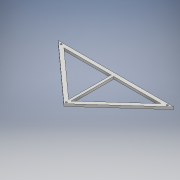
# Autodesk Inventor part: Down base
Saved by Autodesk Inventor 2018 (Build 220112000, 112)
## iProperties
Created: 2019-11-10
Part Number: Down base
Material: Типовые
Document SubType Name: Modeling
Designer: cosko
Density: 1 g/cm^3
Appearance: По умолчанию
Author: cosko
Autodesk Inventor part; units mm, degrees
ref_plane "YZ Plane" through (0, 0, 0) normal (1, 0, 0) x (0, 1, 0)
ref_plane "XZ Plane" through (0, 0, 0) normal (0, 1, 0) x (-1, 0, 0)
ref_plane "XY Plane" through (0, 0, 0) normal (0, 0, 1) x (1, 0, 0)
sketch "Эскиз1" plane through (0, 0, 0) normal (0, 0, 1) x (1, 0, 0)
  line L0 (-100, -100) -> (100, -100)
  line L1 (100, -100) -> (100, 100)
  line L2 (100, 100) -> (-100, 100)
  line L3 (-100, 100) -> (-100, -100)
  line L4 (-100, -100) -> (100, 100) construction
  line L5 (100, -100) -> (-100, 100) construction
  point P0 (0, 0)
  dimension "d0" = 200
  dimension "d1" = 200
  constraints: 12 end point, 2 midpoint, 2 parallel, 1 horizontal, 1 perpendicular
  measures "d0" distance of L2.end L1.end
  measures "d1" distance of L1.end L0.end
extrude "Выдавливание1" add sketch "Эскиз1" along normal blind 3
sketch "Эскиз2" plane through (0, 0, 3) normal (0, 0, 1) x (1, 0, 0)
  line L0 (-100, -100) -> (100, -100) projected
  line L1 (100, -100) -> (100, 100) projected
  line L2 (100, 100) -> (-100, 100) projected
  line L3 (-100, 100) -> (-100, -100) projected
  line L4 (-100, 100) -> (-90, 100) construction
  line L5 (-100, -100) -> (100, -100) construction
  line L6 (100, -100) -> (90, -100) construction
  line L7 (-90, 100) -> (-90, 90) construction
  line L8 (100, 100) -> (-100, 100) construction
  line L9 (-90, 100) -> (-80, 100) construction
  line L10 (90, -100) -> (90, -90) construction
  line L11 (-90, 90) -> (90, 90) construction
  line L12 (90, 90) -> (90, -90) construction
  line L13 (90, -90) -> (-90, -90) construction
  line L14 (-90, -90) -> (-90, 90) construction
  point P0 (0, 0)
  dimension "d4" = 10
  dimension "d5" = 10
  dimension "d6" = 10
  dimension "d7" = 270
  dimension "d8" = 10
  constraints: 18 end point, 3 perpendicular, 2 horizontal, 2 parallel, 2 point on line, 1 vertical
  measures "d4" distance of L2.end L4.end
  measures "d5" distance of L0.end L6.end
  measures "d6" distance of L4.end L7.end
  measures "d8" distance of L6.end L10.end
sketch "Эскиз3" plane through (0, 0, 0) normal (0, 0, -1) x (-1, 0, 0)
  line L0 (-90, -90) -> (90, -90) construction
  line L1 (90, -90) -> (90, 90) construction
  line L2 (90, 90) -> (-90, 90) construction
  line L3 (100, -100) -> (-100, -100) projected
  line L4 (-100, -100) -> (-100, 100) projected
  line L5 (-100, 100) -> (100, 100) projected
  line L6 (100, 100) -> (100, -100) projected
  line L7 (-90, 90) -> (-90, -90) construction
  point P0 (0, 0)
sketch "Эскиз4" plane through (0, 0, 0) normal (0, 0, -1) x (-1, 0, 0)
  line L0 (90, -90) -> (90, 90) construction
  line L1 (-90, -90) -> (90, -90) construction
  line L2 (90, -90) -> (80, -90) construction
  line L3 (80, -90) -> (80, -57.8) construction
  line L4 (80, -57.8) -> (69, -57.8) construction
  line L5 (69, -57.8) -> (69, -90) construction
  line L6 (74.5, -90) -> (74.5, -58.2367) construction
  line L7 (80, -73.9) -> (69, -73.9) construction
  line L8 (74.5, -90) -> (74.5, -82.5) construction
  circle A0 centre (74.5, -82.5) radius 2
  line L9 (74.5, -82.5) -> (74.5, -75) construction
  line L10 (74.5, -75) -> (74.5, -67.5) construction
  circle A1 centre (74.5, -75) radius 2
  circle A2 centre (74.5, -67.5) radius 2
  line L11 (69, -90) -> (38, -90) construction
  line L12 (53.5, -90) -> (53.5, -69.5) construction
  line L13 (27, -90) -> (27, -57.8) construction
  line L14 (27, -57.8) -> (38, -57.8) construction
  line L15 (38, -57.8) -> (38, -90) construction
  line L16 (32.5, -90) -> (32.5, -58.2367) construction
  line L17 (27, -73.9) -> (38, -73.9) construction
  line L18 (32.5, -90) -> (32.5, -82.5) construction
  circle A3 centre (32.5, -82.5) radius 2
  line L19 (32.5, -82.5) -> (32.5, -75) construction
  line L20 (32.5, -75) -> (32.5, -67.5) construction
  circle A4 centre (32.5, -75) radius 2
  circle A5 centre (32.5, -67.5) radius 2
  line L21 (0, 90) -> (0, -90)
  line L22 (-80, -90) -> (-80, -57.8) construction
  line L23 (-80, -57.8) -> (-69, -57.8) construction
  line L24 (-69, -57.8) -> (-69, -90) construction
  line L25 (-74.5, -90) -> (-74.5, -58.2367) construction
  line L26 (-80, -73.9) -> (-69, -73.9) construction
  line L27 (-74.5, -90) -> (-74.5, -82.5) construction
  circle A6 centre (-74.5, -82.5) radius 2
  line L28 (-74.5, -82.5) -> (-74.5, -75) construction
  line L29 (-74.5, -75) -> (-74.5, -67.5) construction
  circle A7 centre (-74.5, -75) radius 2
  circle A8 centre (-74.5, -67.5) radius 2
  line L30 (-69, -90) -> (-38, -90) construction
  line L31 (-53.5, -90) -> (-53.5, -69.5) construction
  line L32 (-27, -90) -> (-27, -57.8) construction
  line L33 (-38, -57.8) -> (-38, -90) construction
  line L34 (-27, -73.9) -> (-38, -73.9) construction
  line L35 (-27, -57.8) -> (-38, -57.8) construction
  line L36 (-32.5, -90) -> (-32.5, -58.2367) construction
  line L37 (-32.5, -90) -> (-32.5, -82.5) construction
  circle A9 centre (-32.5, -82.5) radius 2
  line L38 (-32.5, -82.5) -> (-32.5, -75) construction
  circle A10 centre (-32.5, -75) radius 2
  line L39 (-32.5, -75) -> (-32.5, -67.5) construction
  circle A11 centre (-32.5, -67.5) radius 2
  line L40 (27, -57.8) -> (80, -57.8) construction
  line L41 (80, -57.8) -> (80, -29.8) construction
  line L42 (80, -29.8) -> (27, -29.8) construction
  line L43 (27, -29.8) -> (27, -57.8) construction
  line L44 (-80, -57.8) -> (-69, -57.8) construction
  line L45 (-27, -57.8) -> (-38, -57.8) construction
  line L46 (-27, -57.8) -> (-80, -57.8) construction
  line L47 (-80, -57.8) -> (-80, -29.8) construction
  line L48 (-80, -29.8) -> (-27, -29.8) construction
  line L49 (-27, -29.8) -> (-27, -57.8) construction
  line L50 (80, -57.8) -> (27, -57.8) construction
  line L51 (27, -57.8) -> (27, -49.8) construction
  line L52 (27, -49.8) -> (80, -49.8) construction
  line L53 (80, -49.8) -> (80, -57.8) construction
  line L54 (-27, -57.8) -> (-80, -57.8) construction
  line L55 (-80, -57.8) -> (-80, -49.8) construction
  line L56 (-80, -49.8) -> (-27, -49.8) construction
  line L57 (-27, -49.8) -> (-27, -57.8) construction
  line L58 (27, -49.8) -> (80, -49.8)
  line L59 (80, -49.8) -> (80, -21.8)
  line L60 (80, -21.8) -> (27, -21.8)
  line L61 (27, -21.8) -> (27, -49.8)
  line L62 (-27, -49.8) -> (-80, -49.8)
  line L63 (-80, -49.8) -> (-80, -21.8)
  line L64 (-80, -21.8) -> (-27, -21.8)
  line L65 (-27, -21.8) -> (-27, -49.8)
  line L66 (100, -100) -> (-100, -100) construction
  line L67 (100, 100) -> (100, -100) construction
  line L68 (-100, 100) -> (100, 100) construction
  line L69 (-100, -100) -> (-100, 100) construction
  line L70 (-100, -100) -> (-100, 100) construction
  line L71 (-100, -10.3933) -> (-30.663, -10.3933) construction
  line L72 (100, -100) -> (-100, -100) construction
  line L73 (-16.2396, -100) -> (-16.2396, -14.621) construction
  line L74 (-100, 100) -> (100, 100) construction
  line L75 (-16.2396, 100) -> (-16.2396, -4.35) construction
  line L76 (-16.2396, 100) -> (88.1104, 100) construction
  line L77 (-30.663, -4.35) -> (-30.663, -14.621)
  line L78 (-30.663, -9.4855) -> (-27.663, -9.4855) construction
  line L79 (-27.663, -4.35) -> (-27.663, -14.621) construction
  line L80 (-30.663, -14.621) -> (-16.2396, -14.621) construction
  line L81 (-30.663, -4.35) -> (-16.2396, -4.35) construction
  line L82 (-16.2396, -14.621) -> (-16.2396, -4.35) construction
  line L83 (-27.663, -14.621) -> (-27.663, -12.053) construction
  circle A12 centre (-27.663, -12.053) radius 1.5
  line L84 (-27.663, -12.053) -> (-27.663, -6.918) construction
  circle A13 centre (-27.663, -6.918) radius 1.5
  line L85 (-30.663, -10.3933) -> (-53.163, -10.3933) construction
  line L86 (-30.663, -4.35) -> (-30.663, 18.15) construction
  line L87 (-30.663, 6.9) -> (-19.0358, 6.9) construction
  line L88 (-30.663, 18.15) -> (-30.663, 28.421)
  line L89 (-30.663, 23.2855) -> (-27.663, 23.2855) construction
  line L90 (-27.663, 18.15) -> (-27.663, 28.421) construction
  line L91 (-27.663, 28.421) -> (-27.663, 25.853) construction
  circle A14 centre (-27.663, 25.853) radius 1.5
  line L92 (-27.663, 25.853) -> (-27.663, 20.718) construction
  circle A15 centre (-27.663, 20.718) radius 1.5
  line L93 (-30.663, 28.421) -> (29.337, 28.421) construction
  line L94 (29.337, 28.421) -> (29.337, -14.621) construction
  line L95 (29.337, -14.621) -> (-30.663, -14.621) construction
  line L96 (-30.663, -14.621) -> (-30.663, 28.421) construction
  line L97 (-30.663, 28.421) -> (29.337, -14.621) construction
  line L98 (29.337, 28.421) -> (-30.663, -14.621) construction
  line L99 (-32.163, -16.1) -> (30.837, -16.1) construction
  line L100 (30.837, -16.1) -> (30.837, 29.9) construction
  line L101 (30.837, 29.9) -> (-32.163, 29.9) construction
  line L102 (-32.163, 29.9) -> (-32.163, -16.1) construction
  line L103 (-32.163, -16.1) -> (30.837, 29.9) construction
  line L104 (30.837, -16.1) -> (-32.163, 29.9) construction
  line L105 (-100, -21.8) -> (100, -21.8) construction
  line L106 (100, -21.8) -> (100, 29.9) construction
  line L107 (100, 29.9) -> (-100, 29.9) construction
  line L108 (-100, 29.9) -> (-100, -21.8) construction
  line L109 (100, 100) -> (100, -100) construction
  line L110 (100, 4.05) -> (-100, 4.05) construction
  line L111 (-90, -90) -> (-90, 47.825) construction
  line L112 (90, -21.8) -> (90, 4.05) construction
  line L113 (-90, -21.0875) -> (-90, 4.05) construction
  line L114 (-90, -8.5187) -> (90, -8.875) construction
  circle A16 centre (-90, -8.5187) radius 1.5
  circle A17 centre (90, -8.875) radius 1.5
  circle A18 centre (0, -90) radius 1.5
  line L115 (100, 4.05) -> (30.837, 4.05) construction
  line L116 (30.837, 4.05) -> (30.837, 100) construction
  line L117 (30.837, 100) -> (100, 100) construction
  line L118 (100, 100) -> (100, 4.05) construction
  line L119 (30.837, 4.05) -> (100, 4.05)
  line L120 (100, 4.05) -> (100, 100)
  line L121 (100, 100) -> (30.837, 100)
  line L122 (30.837, 100) -> (30.837, 4.05)
  line L123 (30.837, 100) -> (-100, 100)
  line L124 (-100, 100) -> (-100, 29.9)
  line L125 (-100, 29.9) -> (30.837, 29.9)
  line L126 (30.837, 29.9) -> (30.837, 100)
  line L127 (-100, 29.9) -> (-32.163, 29.9)
  line L128 (-32.163, 29.9) -> (-32.163, 4.05)
  line L129 (-32.163, 4.05) -> (-100, 4.05)
  line L130 (-100, 4.05) -> (-100, 29.9)
  line L131 (0, -8.6969) -> (-5, -8.6969) construction
  line L132 (0, -8.6969) -> (5, -8.6969) construction
  line L133 (90, -90) -> (100, -80)
  line L134 (90, -90) -> (104.1421, -90) construction
  line L135 (100, -80) -> (80, -100)
  line L136 (100, -100) -> (-100, -100) projected
  line L137 (80, -100) -> (100, -100)
  line L138 (100, -100) -> (100, -80)
  line L139 (-100, -100) -> (100, -100) construction
  line L140 (-100, -100) -> (100, -100) construction
  line L141 (-100, -80) -> (-80, -100)
  line L142 (-100, -100) -> (100, -100)
  line L143 (-100, -100) -> (-100, -80)
  line L144 (100, 100) -> (100, -100) projected
  line L145 (100, -21.8) -> (87.631, -21.8) construction
  line L146 (87.631, 4.05) -> (87.631, -19.5) construction
  line L147 (87.631, -21.8) -> (87.631, -18.7327) construction
  circle A19 centre (87.631, -19.5) radius 2
  line L148 (87.631, -19.5) -> (97.631, -19.5) construction
  circle A20 centre (97.631, -19.5) radius 2
  line L149 (87.631, -19.5) -> (87.631, -53.5) construction
  line L150 (87.631, -36.5) -> (80, -36.5) construction
  circle A21 centre (87.631, -53.5) radius 2
  line L151 (87.631, -53.5) -> (97.631, -53.5) construction
  circle A22 centre (97.631, -53.5) radius 2
  circle A23 centre (-87.631, -19.5) radius 2
  line L152 (-87.631, -19.5) -> (-97.631, -19.5) construction
  circle A24 centre (-97.631, -19.5) radius 2
  circle A25 centre (-87.631, -53.5) radius 2
  line L153 (-87.631, -53.5) -> (-97.631, -53.5) construction
  circle A26 centre (-97.631, -53.5) radius 2
  point P0 (0, 0)
  point P1 (-30.663, 24.1933)
  point P2 (-0.663, 6.9)
  dimension "d9" = 10
  dimension "d10" = 32.2
  dimension "d11" = 11
  dimension "d12" = 7.5
  dimension "d13" = 4
  dimension "d14" = 7.5
  dimension "d15" = 7.5
  dimension "d16" = 4
  dimension "d17" = 4
  dimension "d18" = 31
  dimension "d23" = 28
  dimension "d24" = 8
  dimension "d25" = 8
  dimension "d26" = 28
  dimension "d27" = 28
  dimension "d31" = 69.337
  dimension "d32" = 85.379
  dimension "d33" = 104.35
  dimension "d34" = 90
  dimension "d35" = 3
  dimension "d36" = 2.568
  dimension "d37" = 3
  dimension "d38" = 5.135
  dimension "d39" = 3
  dimension "d40" = 22.5
  dimension "d41" = 22.5
  dimension "d44" = 60
  dimension "d45" = 63
  dimension "d46" = 46
  dimension "d47" = 3
  dimension "d48" = 3
  dimension "d49" = 3
  dimension "d54" = 5
  dimension "d55" = 180
  dimension "d59" = 45
  dimension "d62" = 12.369
  dimension "d63" = 23.55
  dimension "d64" = 4
  dimension "d65" = 10
  dimension "d66" = 4
  dimension "d67" = 34
  constraints: 284 end point, 71 symmetric about line, 46 point on line, 27 centre point, 26 parallel, 25 coincident, 23 horizontal, 19 perpendicular, 15 midpoint, 7 vertical, 3 equal length, 18 other
  measures "d9" distance of L0.start L2.end
  measures "d10" distance of L2.end L3.end
  measures "d11" distance of L3.end L4.end
  measures "d12" distance of L6.start L8.end
  measures "d13" diameter of A0
  measures "d14" distance of L9.start L9.end
  measures "d15" distance of L9.end L10.end
  measures "d16" diameter of A1
  measures "d17" diameter of A2
  measures "d18" distance of L5.end L11.end
  measures "d23" distance of L41.end L40.end
  measures "d24" distance of L50.end L51.end
  measures "d25" distance of L54.end L55.end
  measures "d26" distance of L59.end L58.end
  measures "d27" distance of L62.end L63.end
  measures "d31" distance of L71.start L71.end
  measures "d32" distance of L73.start L73.end
  measures "d33" distance of L75.start L75.end
  measures "d34" angle of L75 L76
  measures "d35" distance of L78.start L78.end
  measures "d36" distance of L79.end L83.end
  measures "d37" diameter of A12
  measures "d38" distance of L84.start L84.end
  measures "d39" diameter of A13
  measures "d40" distance of L71.end L85.end
  measures "d41" distance of L77.start L86.end
  measures "d44" distance of L94.end L95.end
  measures "d45" distance of L101.end L100.end
  measures "d46" distance of L100.end L99.end
  measures "d47" diameter of A16
  measures "d48" diameter of A17
  measures "d49" diameter of A18
  measures "d54" distance of L131.start L131.end
  measures "d55" angle of L131 L132
  measures "d59" angle of L134 L133
  measures "d62" distance of L105.end L145.end
  measures "d63" distance of L146.start L146.end
  measures "d64" diameter of A19
  measures "d65" distance of L148.start L148.end
  measures "d66" diameter of A20
  measures "d67" distance of L148.start L149.end
extrude "Выдавливание2" cut sketch "Эскиз4" against normal blind 10 contours A0 | A1 | A2 | A3 | A4 | A5
extrude "Выдавливание3" cut sketch "Эскиз4" against normal blind 10 contours A6 | A7 | A8 | A9 | A10 | A11
extrude "Выдавливание4" cut sketch "Эскиз4" against normal blind 10 contours L61 L60 L59 L58 | L62 L63 L64 L65
extrude "Выдавливание5" cut sketch "Эскиз4" against normal blind 10 contours A12 | A13 | A14 | A15
extrude "Выдавливание6" cut sketch "Эскиз4" against normal blind 10 contours A18 | A16 | A17
extrude "Выдавливание7" cut sketch "Эскиз4" against normal blind 10 contours L125 L124 L123 L122 | L128 L129 L130 L125 | L122 L121 L120 L119
extrude "Выдавливание9" cut sketch "Эскиз4" against normal blind 10 contours L136 L143 L141 | L138 L136 L135 L133
extrude "Выдавливание10" cut sketch "Эскиз4" against normal blind 10 contours A19 | A20 | A21 | A22 | A23 | A24 | A25 | A26
sketch "Эскиз5" plane through (0, 0, 3) normal (0, 0, 1) x (1, 0, 0)
  circle A0 centre (-90, -8.875) radius 1.5 projected
  circle A1 centre (90, -8.5187) radius 1.5 projected
  circle A2 centre (0, -90) radius 1.5 projected
  line L0 (-90, -8.875) -> (90, -8.5187) construction
  circle A3 centre (0, -90) radius 1.5 construction
  line L1 (90, -8.5187) -> (0, -90) construction
  line L2 (0, -90) -> (-90, -8.875) construction
  line L3 (-82.2082, -11.8596) -> (-2.1284, -84.0426)
  line L4 (2.1196, -84.0342) -> (82.1994, -11.5342)
  line L5 (-97.7918, -5.8904) -> (0.0044, -94.0428)
  line L6 (0.0044, -94.0428) -> (97.8006, -5.5033)
  line L7 (-0.0044, -11.6969) -> (-0.0044, -85.9572) construction
  line L8 (2.1196, -5.6927) -> (-2.1284, -5.6927)
  line L9 (2.1196, -84.0342) -> (2.1196, -11.6927)
  line L10 (1.7459, -84.3725) -> (-1.8325, -11.7005) construction
  line L11 (-2.128, -5.7011) -> (-2.1284, -5.6927) construction
  line L12 (-2.1284, -5.6927) -> (-2.1284, -5.7011)
  line L13 (97.8006, -5.5033) -> (2.1196, -5.6927)
  line L14 (-2.128, -5.7011) -> (-97.7918, -5.8904)
  line L15 (-2.1284, -11.7011) -> (-2.1284, -84.0426)
  line L16 (-2.1284, -91.9269) -> (-2.1284, -91.9614)
  line L17 (-2.1284, -91.9614) -> (-2.1266, -91.9253) construction
  line L18 (-1.755, -84.3792) -> (1.8241, -11.6933) construction
  line L19 (82.1994, -11.5342) -> (2.1196, -11.6927)
  line L20 (-2.1284, -11.7011) -> (-82.2082, -11.8596)
  point P0 (0, 0)
  point P1 (-0.0044, -48.827)
  constraints: 42 end point, 5 point on line, 3 parallel, 1 midpoint, 1 vertical, 1 other
extrude "Выдавливание11" add sketch "Эскиз5" along normal blind 4 separate body
